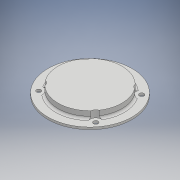
# Autodesk Inventor part: FilterHolderSmall
Saved by Autodesk Inventor 2017 (Build 210142000, 142)
## iProperties
Created: 2017-12-06
Part Number: FilterHolderSmall
Material: Generic
Document SubType Name: Modeling
Designer: Paolo
Density: 1 g/cm^3
Appearance: Default
Author: Paolo
Autodesk Inventor part; units mm, degrees
ref_plane "YZ Plane" through (0, 0, 0) normal (1, 0, 0) x (0, 1, 0)
ref_plane "XZ Plane" through (0, 0, 0) normal (0, 1, 0) x (-1, 0, 0)
ref_plane "XY Plane" through (0, 0, 0) normal (0, 0, 1) x (1, 0, 0)
sketch "Sketch1" plane through (0, 0, 0) normal (0, 0, 1) x (1, 0, 0)
  circle A0 centre (0, 0) radius 12.7 projected
  circle A1 centre (0, 0) radius 10.5 projected
  circle A2 centre (0, 0) radius 14.3
  dimension "d0" = 1.6
  constraints: 1 centre point
  measures "d0" radial gap between concentric circles of A0 A2
extrude "Extrusion1" add sketch "Sketch1" along normal blind 1.6 contours A0 | A2
sketch "Sketch2" plane through (0, 0, 0) normal (0, 0, -1) x (-1, 0, 0)
  circle A0 centre (0, 0) radius 12.7 projected
  circle A1 centre (0, 0) radius 14.3 projected
  circle A2 centre (0, 0) radius 13
  dimension "d3" = 0.3
  constraints: 1 centre point
  measures "d3" radial gap between concentric circles of A0 A2
extrude "Extrusion2" add sketch "Sketch2" along normal blind 6.3 contours A1
sketch "Sketch3" plane through (0, 0, -6.3) normal (0, 0, -1) x (-1, 0, 0)
  circle A0 centre (0, 0) radius 14.3 projected
  circle A1 centre (19.8743, -0.3764) radius 1.05 projected
  circle A2 centre (12.6657, 10.2607) radius 1 projected
  circle A3 centre (-12.3285, 10.8) radius 1.05 projected
  circle A4 centre (-20.1164, 0.4865) radius 1.05 projected
  circle A5 centre (-12.7815, -10.1951) radius 1.05 projected
  circle A6 centre (12.2127, -10.7344) radius 1 projected
  circle A7 centre (0, 0) radius 18.8
  circle A8 centre (0, 0) radius 13 projected
  dimension "d6" = 4.5
  constraints: 1 centre point
  measures "d6" radial gap between concentric circles of A0 A7
ref_plane "Work Plane1" through (-47.7309, -37.9502, -7.3) normal (0, 0, 1) x (0.9997673, 0.0215719, 0)
extrude "Extrusion3" add sketch "Sketch3" along normal up to surface (1 mm away) contours A0 | A7
fillet "Fillet1" radius 1 1 edges at (14.3, 0, -6.3)
sketch "Sketch4" plane through (0, 0, -6.3) normal (0, 0, 1) x (1, 0, 0)
  arc A0 (-11.6701, -9.8944) -> (-11.31, -10.3041) centre (-12.2127, -10.7344) ccw projected
  circle A1 centre (-12.2127, -10.7344) radius 2.5
  circle A2 centre (12.7815, -10.1951) radius 1.05 projected
  circle A3 centre (12.7815, -10.1951) radius 2.5
  circle A4 centre (12.3285, 10.8) radius 1.05 projected
  circle A5 centre (12.3285, 10.8) radius 2.5
  circle A6 centre (-12.6657, 10.2607) radius 1 projected
  circle A7 centre (-12.6657, 10.2607) radius 2.5
  circle A8 centre (-12.2127, -10.7344) radius 1
  point P0 (0, 0)
  dimension "d10" = 5
  dimension "d11" = 5
  dimension "d12" = 5
  dimension "d13" = 5
  constraints: 5 centre point, 5 coincident, 1 concentric
  measures "d10" diameter of A1
  measures "d11" diameter of A3
  measures "d12" diameter of A5
  measures "d13" diameter of A7
extrude "Extrusion4" cut sketch "Sketch4" along normal blind 8.05
move faces "Move1" translate (0, 0, -3) faces at (11.3639, 6.2368, 1.6)
move faces "Move2" translate (0, 0, -3.25) faces at (-12.4731, -4.8138, -1.4)
sketch "Sketch5" plane through (0, 0, -4.65) normal (0, 0, 1) x (0.9998882, 0.0149516, 0)
  circle A0 centre (0, 0) radius 13 projected
  arc A1 (10.0233, 10.1991) -> (11.6814, 8.2484) centre (12.4886, 10.6144) ccw projected
  arc A2 (10.0233, 10.1991) -> (-10.0233, 10.1991) centre (0, 0) ccw projected
  arc A3 (-11.8219, 8.0457) -> (-10.0233, 10.1991) centre (-12.5108, 10.4489) ccw projected
  arc A4 (-11.8219, 8.0457) -> (-11.7677, -8.1247) centre (0, 0) ccw projected
  arc A5 (-9.8809, -10.3372) -> (-11.7677, -8.1247) centre (-12.3718, -10.5506) ccw projected
  arc A6 (-9.8809, -10.3372) -> (10.1468, -10.0763) centre (0, 0) ccw projected
  arc A7 (11.8457, -8.0105) -> (10.1468, -10.0763) centre (12.6277, -10.3851) ccw projected
  arc A8 (11.8457, -8.0105) -> (11.6814, 8.2484) centre (0, 0) ccw projected
extrude "Extrusion5" add sketch "Sketch5" along normal blind 1.5 contours A0 | A1 A8 A7 A6 A5 A4 A3 A2
sketch "Sketch6" plane through (0, 0, -4.65) normal (0, 0, -1) x (-1, 0, 0)
  circle A0 centre (0, 0) radius 13 projected
  point P0 (0, 0)
body "Solid1"
